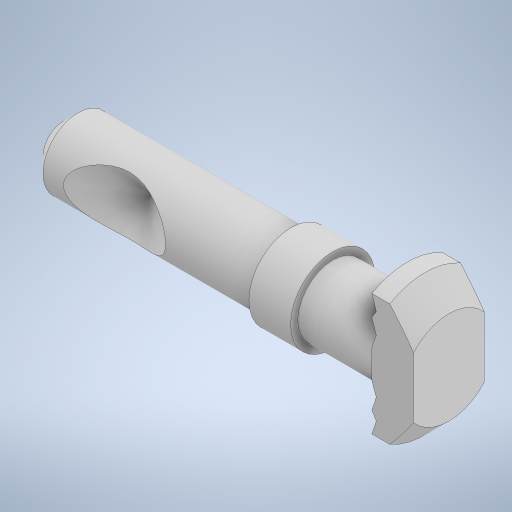
# Autodesk Inventor part: Tornillo en T esquinero
Saved by Autodesk Inventor 2024.2 (Build 282272000, 272)
## iProperties
Created: 2025-07-16
Part Number: Tornillo en T esquinero
Material: Generic
Document SubType Name: Modeling
Designer: ja.restrepo1
Density: 1 g/cm^3
Appearance: Default
Author: ja.restrepo1
Autodesk Inventor part; units mm, degrees
ref_plane "YZ Plane" through (0, 0, 0) normal (1, 0, 0) x (0, 1, 0)
sketch "Sketch1" plane through (0, 0, 0) normal (0, 0, 1) x (1, 0, 0)
  line L0 (25.9, 0) -> (25.9, 6.25)
  line L1 (22.7, 9.45) -> (20.3, 9.45)
  line L2 (20.3, 9.45) -> (20.3, 7.175) construction
  line L3 (20.3, 4.7) -> (10.3, 4.7)
  line L4 (10.3, 4.7) -> (10.3, 5.65)
  line L5 (10.3, 5.65) -> (4.7, 5.65)
  line L6 (4.7, 5.65) -> (4.7, 4.7)
  line L7 (4.7, 4.7) -> (-23.9, 4.7)
  line L8 (-25.9, 2.7) -> (-25.9, 0)
  line L9 (-25.9, 0) -> (25.9, 0)
  line L10 (-23.9, 4.7) -> (-25.9, 2.7)
  line L11 (25.9, 6.25) -> (22.7, 9.45)
  line L12 (20.3, 9.45) -> (20.9, 7.95)
  line L13 (20.9, 7.95) -> (20.3, 7.175)
  line L14 (20.3, 7.175) -> (20.9, 5.95)
  line L15 (20.9, 5.95) -> (20.3, 5.1)
  line L16 (20.3, 7.175) -> (20.3, 5.1) construction
  line L17 (20.3, 5.1) -> (20.3, 4.7)
  point P0 (0, 0)
  point P1 (25.9, 9.45)
  point P2 (-25.9, 4.7)
  point P3 (0, 0)
  dimension "d0" = 9.45
  dimension "d1" = 5.6
  dimension "d2" = 51.8
  dimension "d3" = 4.7
  dimension "d4" = 10
  dimension "d5" = 5.6
  dimension "d6" = 5.65
  dimension "d7" = 2
  dimension "d8" = 2
  dimension "d10" = 3.2
  dimension "d11" = 3.2
  dimension "d26" = 0.6
  dimension "d27" = 1.5
  dimension "d28" = 2
  dimension "d29" = 0.4
  dimension "d30" = 2.275
  constraints: 36 end point, 12 perpendicular, 7 point on line, 2 coincident, 1 midpoint, 1 vertical, 1 vertical alignment
  measures "d0" distance of L0.start point (25.9, 9.45)
  measures "d1" distance of point (25.9, 9.45) L1.end
  measures "d2" distance of L8.end L0.start
  measures "d3" distance between parallel lines of L3 L9
  measures "d4" distance of L3.start L3.end
  measures "d5" distance of L4.end L5.end
  measures "d6" distance between parallel lines of L5 L9
  measures "d7" distance of L7.end point (-25.9, 4.7)
  measures "d8" distance of L8.start point (-25.9, 4.7)
  measures "d10" distance of L0.end point (25.9, 9.45)
  measures "d11" distance of L1.start point (25.9, 9.45)
  measures "d26" distance from line of L12.end L2
  measures "d27" distance from line of L12.end L1
  measures "d28" distance of L14.end L12.end
  measures "d29" distance of L3.start L15.end
  measures "d30" distance from line of L1 L2.end
revolve "Revolution1" add sketch "Sketch1" angle 360 about axis through (-25.9, 0, 0) along (1, 0, 0)
sketch "Sketch2" plane through (25.9, 0, 0) normal (1, 0, 0) x (0, 0, -1)
  line L0 (-4.75, 9.5) -> (4.75, 9.5) construction
  line L1 (4.75, 9.5) -> (4.75, -9.5)
  line L2 (4.75, -9.5) -> (-4.75, -9.5) construction
  line L3 (-4.75, -9.5) -> (-4.75, 9.5)
  line L4 (4.75, 9.5) -> (9.75, 9.5)
  line L5 (9.75, 9.5) -> (9.75, -9.5)
  line L6 (9.75, -9.5) -> (4.75, -9.5)
  line L7 (-4.75, 9.5) -> (-9.75, 9.5)
  line L8 (-9.75, 9.5) -> (-9.75, -9.5)
  line L9 (-9.75, -9.5) -> (-4.75, -9.5)
  point P0 (0, 0)
  point P1 (0, 9.5)
  point P2 (-4.75, 0)
  dimension "d12" = 9.5
  dimension "d13" = 19
  dimension "d14" = 5
  constraints: 20 end point, 5 perpendicular, 3 horizontal, 2 midpoint, 2 parallel, 1 collinear, 1 horizontal alignment, 1 vertical alignment
  measures "d12" distance of L0.start L0.end
  measures "d13" distance of L0.end L1.end
  measures "d14" distance of L5.end L1.end
extrude "Extrusion1" cut sketch "Sketch2" against normal blind 5.8
ref_plane "Work Plane1" through (0, 4.9, 0) normal (0, 1, 0) x (-1, 0, 0)
sketch "Sketch3" plane through (0, 4.9, 0) normal (0, 1, 0) x (-1, 0, 0)
  line L0 (-4.7, 5.65) -> (-4.7, -5.65) projected
  point P0 (0, 0)
  point P1 (14.3, 0)
  dimension "d18" = 19
  constraints: 1 horizontal alignment
  measures "d18" distance from line of point (14.3, 0) L0
hole "0°" [suppressed]
ref_plane "Work Plane2" through (0, 0, 5) normal (0, 0, 1) x (1, 0, 0)
sketch "Sketch4" plane through (0, 0, 5) normal (0, 0, 1) x (1, 0, 0)
  line L0 (4.7, -5.65) -> (4.7, 5.65) projected
  point P0 (0, 0)
  point P1 (-14.3, 0)
  dimension "d32" = 19
  constraints: 1 horizontal alignment
  measures "d32" distance from line of point (-14.3, 0) L0
hole "90°" at (-14.3, 0, 5) direction (0, 0, -1) diameter 14 depth 0.2 tip angle 110
equation "\"d8\" = d7"
equation "\"d11\" = d10"
body "Solid1"
